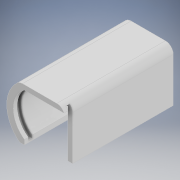
# Autodesk Inventor part: Case_Side
Saved by Autodesk Inventor 2020 (Build 240168000, 168)
## iProperties
Created: 2019-11-07
Part Number: Case_Side
Material: 일반
Document SubType Name: Modeling
Designer: Knowblesse
Density: 1 g/cm^3
Appearance: 기본값
Author: Knowblesse
## iProperties of the stored document _3D 인쇄.ipt
Created: 2020-02-25
Part Number: _3D 인쇄
Material: 일반
Document SubType Name: Modeling
Designer: Knowblesse
Density: 1 g/cm^3
Appearance: 기본값
Author: Knowblesse
Autodesk Inventor part; units mm, degrees
ref_plane "YZ Plane" through (0, 0, 0) normal (1, 0, 0) x (0, 1, 0)
ref_plane "XZ Plane" through (0, 0, 0) normal (0, 1, 0) x (-1, 0, 0)
ref_plane "XY Plane" through (0, 0, 0) normal (0, 0, 1) x (1, 0, 0)
sketch "스케치1" plane through (0, 0, 0) normal (0, 0, 1) x (1, 0, 0)
  line L0 (0, 0) -> (9, 0)
  line L1 (9, 0) -> (9, 10.8)
  line L2 (9, 10.8) -> (0, 10.8)
  line L3 (0, 10.8) -> (0, 0)
  line L4 (-1.2, 12) -> (10.2, 12)
  line L5 (10.2, 12) -> (10.2, -1.2)
  line L6 (10.2, -1.2) -> (-1.2, -1.2)
  line L7 (-1.2, -1.2) -> (-1.2, 12)
  line L8 (0, 0) -> (0, -1.2)
  line L9 (9, 0) -> (9, -1.2)
  line L10 (0, 0) -> (-1.2, 0)
  line L11 (9, 0) -> (10.2, 0)
  arc A0 (-1.2, 12) -> (-1.2, -1.2) centre (3.7811, 5.4) ccw
  arc A1 (0, 10.8) -> (0, 0) centre (3.7811, 5.4) ccw
  line L12 (-1.2, 10.4) -> (0, 10.4) construction
  line L13 (0, 10.4) -> (0, 0.4) construction
  line L14 (0, 0.4) -> (-1.2, 0.4) construction
  line L15 (-1.2, 0.4) -> (-1.2, 10.4) construction
  point P0 (0, 5.4)
  dimension "d0" = 9
  dimension "d1" = 10.8
  dimension "d2" = 1.2
  dimension "d35" = 10
  dimension "d36" = 110
  constraints: 32 end point, 8 point on line, 6 parallel, 5 perpendicular, 4 point on circle, 2 centre point, 2 horizontal, 2 midpoint, 1 concentric, 3 other
  measures "d0" distance of L2.end L1.end
  measures "d1" distance of L1.end L0.end
  measures "d2" distance between parallel lines of L2 L4
  measures "d35" distance between parallel lines of L14 L12
extrude "돌출1" add sketch "스케치1" along normal blind 20 contours L8 L6 L7 L10 | L10 L7 A1 | L11 L5 L6 L9 | L1 L2 A1 L7 L4 L5 L11 | L7 A0 A1
sketch "스케치5" plane through (0, 10.8, 0) normal (0, -1, 0) x (1, 0, 0)
  line L0 (0, 0) -> (9, 0) projected
  line L1 (9, 0) -> (9, 20) projected
  line L2 (0, 20) -> (9, 20) projected
  line L3 (0, 0) -> (0, 20) projected
  line L4 (9, 17.5) -> (7, 17.5)
  line L5 (7, 17.5) -> (7, 20)
  line L6 (10.2, 20) -> (-1.2, 20) projected
  point P0 (0, 0)
  point P1 (8.2, 20)
  point P2 (-0.4776, 20)
  dimension "d21" = 2.5
  dimension "d22" = 2
  constraints: 4 end point, 2 point on line, 1 horizontal, 1 perpendicular
  measures "d21" distance between parallel lines of L2 L4
  measures "d22" distance between parallel lines of L5 L1
extrude "돌출5" add sketch "스케치5" along normal blind 5 contours L4 L5 L2 L1
sketch "스케치8" plane through (0, -1.2, 0) normal (1, 0, 0) x (0, 0, -1)
  line L0 (0, 0) -> (-20, 0) projected
  line L1 (0, 0) -> (0, 1.2) projected
  line L2 (0, 0) -> (-20, 0) projected
  line L3 (-5, 0) -> (-5.8, 0)
  line L4 (-5.8, 0) -> (-5.8, 8)
  line L5 (-5.8, 8) -> (-5, 8)
  line L6 (-5, 8) -> (-5, 0)
  point P0 (-18.5, 0)
  point P1 (-5.8, 0)
  point P2 (-5, 0)
  dimension "d37" = 5
  dimension "d38" = 0.8
  dimension "d39" = 8
  constraints: 8 end point, 2 parallel, 1 horizontal, 1 perpendicular, 1 point on line
  measures "d37" distance between parallel lines of L6 L1
  measures "d38" distance between parallel lines of L4 L6
  measures "d39" distance between parallel lines of L0 L5
extrude "돌출7" cut sketch "스케치8" against normal through all
sketch "스케치13" plane through (0, 0, 20) normal (0, 0, 1) x (1, 0, 0)
  line L0 (0, 10.8) -> (7, 10.8) projected
  line L1 (9, 5.8) -> (9, -1.2) projected
  line L2 (9, -1.2) -> (10.2, -1.2) projected
  line L3 (10.2, -1.2) -> (10.2, 12) projected
  line L4 (10.2, 12) -> (-1.2, 12) projected
  arc A0 (-1.2, 12) -> (-1.2, -1.2) centre (3.7811, 5.4) ccw projected
  line L5 (-1.2, -1.2) -> (0, -1.2) projected
  line L6 (0, -1.2) -> (0, 0) projected
  arc A1 (0, 10.8) -> (0, 0) centre (3.7811, 5.4) ccw projected
  line L7 (0, 10.8) -> (9, 10.8) projected
  line L8 (7, 10.8) -> (9, 10.8)
  line L9 (9, 10.8) -> (9, 5.8)
  constraints: 4 end point, 1 horizontal, 1 perpendicular
extrude "돌출11" add sketch "스케치13" along normal blind 5.5
sketch "스케치14" plane through (0, 0, 25.5) normal (0, 0, 1) x (1, 0, 0)
  line L0 (10.2, -1.2) -> (10.2, 12) projected
  line L1 (10.2, 12) -> (-1.2, 12) projected
  arc A0 (-1.2, 12) -> (-1.2, -1.2) centre (3.7811, 5.4) ccw projected
  line L2 (-1.2, -1.2) -> (0, -1.2) projected
  line L3 (0, -1.2) -> (0, 0) projected
  arc A1 (0, 10.8) -> (0, 0) centre (3.7811, 5.4) ccw projected
  line L4 (0, 10.8) -> (9, 10.8) projected
  arc A2 (-0.8195, 11.55) -> (-0.8195, -0.75) centre (4.7076, 5.4) ccw
  line L5 (-0.8195, 11.55) -> (10.2, 11.55)
  line L6 (10.2, -1.2) -> (10.2, 12) projected
  line L7 (-0.8195, -0.75) -> (0, -0.75)
  dimension "d53" = 0.75
  dimension "d55" = 0.75
  dimension "d56" = 0.75
  constraints: 4 end point, 2 perpendicular, 2 point on circle, 2 point on line, 1 centre point, 1 equal radius, 1 horizontal alignment
  measures "d53" distance between parallel lines of L4 L5
  measures "d55" distance from line of L3.end L7
extrude "돌출12" add sketch "스케치14" along normal blind 1
sketch "스케치15" plane through (0, 0, 26.5) normal (0, 0, 1) x (1, 0, 0)
  line L0 (10.2, 11.55) -> (10.2, 12) projected
  line L1 (10.2, 12) -> (-1.2, 12) projected
  arc A0 (-1.2, 12) -> (-1.2, -1.2) centre (3.7811, 5.4) ccw projected
  line L2 (-1.2, -1.2) -> (0, -1.2) projected
  line L3 (0, -1.2) -> (0, -0.75) projected
  line L4 (10.2, 11.55) -> (-0.8195, 11.55) projected
  arc A1 (-0.8195, 11.55) -> (-0.8195, -0.75) centre (4.7076, 5.4) ccw projected
  line L5 (-0.8195, -0.75) -> (0, -0.75) projected
  line L6 (0, -0.75) -> (0, 0) projected
  arc A2 (0, 10.8) -> (0, 0) centre (3.7811, 5.4) ccw projected
  line L7 (0, 10.8) -> (9, 10.8) projected
  line L8 (9, 10.8) -> (9, -1.2) projected
  line L9 (9, -1.2) -> (10.2, -1.2) projected
  line L10 (10.2, -1.2) -> (10.2, 11.55) projected
  line L11 (9, 10.8) -> (10.2, 10.8)
  constraints: 2 end point, 1 perpendicular, 1 point on line
extrude "돌출13" add sketch "스케치15" along normal blind 1 contours L4 A1 L5 L3 L2 A0 L1 L0 | L10 L11 L7 A2 L6 L5 A1 L4
fillet "모깎기2" radius 2 2 edges at (10.2, 12, 13.75) (-1.2, 12, 13.75)
equation "\"d56\" = d55"
